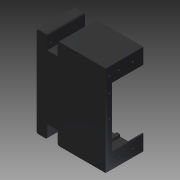
# Autodesk Inventor part: Part1
Saved by Autodesk Inventor 2016 (Build 200138000, 138)
## iProperties
Created: 2015-06-07
Part Number: Part1
Material: ABS Plastic
Document SubType Name: Modeling
Designer: Jufo
Density: 1 g/cm^3
Appearance: Smooth - White
Author: Jufo
Autodesk Inventor part; units mm, degrees
ref_plane "YZ Plane" through (0, 0, 0) normal (1, 0, 0) x (0, 1, 0)
ref_plane "XZ Plane" through (0, 0, 0) normal (0, 1, 0) x (-1, 0, 0)
ref_plane "XY Plane" through (0, 0, 0) normal (0, 0, 1) x (1, 0, 0)
sketch "Sketch1" plane through (0, 0, 0) normal (0, 1, 0) x (-1, 0, 0)
  line L0 (-6.278, 25.2242) -> (-6.278, -144.7758)
  line L1 (-6.278, -144.7758) -> (-26.278, -144.7758)
  line L2 (-26.278, -144.7758) -> (-26.278, -119.7758)
  line L3 (-26.278, -119.7758) -> (-46.278, -119.7758)
  line L4 (-46.278, -119.7758) -> (-46.278, -144.7758)
  line L5 (-46.278, -144.7758) -> (-136.278, -144.7758)
  line L6 (-136.278, -144.7758) -> (-136.278, -134.7758)
  line L7 (-6.278, 25.2242) -> (-26.278, 25.2242)
  line L8 (-26.278, 25.2242) -> (-26.278, 0.2242)
  line L9 (-26.278, 0.2242) -> (-46.278, 0.2242)
  line L10 (-46.278, 0.2242) -> (-46.278, 25.2242)
  line L11 (-46.278, 25.2242) -> (-136.278, 25.2242)
  line L12 (-136.278, 25.2242) -> (-136.278, 15.2242)
  line L13 (-136.278, 15.2242) -> (-136.278, -134.7758)
  point P0 (0, 0)
  dimension "d0" = 170
  dimension "d1" = 20
  dimension "d3" = 20
  dimension "d4" = 90
  dimension "d80" = 20
  dimension "d81" = 150
  dimension "d82" = 10
  dimension "d83" = 10
  dimension "d84" = 90
  dimension "d226" = 25
  dimension "d227" = 25
  dimension "d228" = 25
  constraints: 28 end point, 10 perpendicular, 3 parallel, 1 vertical
  measures "d0" distance of L0.start L0.end
  measures "d1" distance of L0.end L1.end
  measures "d3" distance of L2.end L3.end
  measures "d4" distance of L4.end L5.end
  measures "d80" distance of L0.start L8.start
  measures "d81" distance of L12.end L6.end
  measures "d82" distance of L12.start L12.end
  measures "d83" distance of L5.end L6.end
  measures "d84" distance of L11.start L12.start
  measures "d226" distance of L10.start L11.start
  measures "d227" distance of L3.end L4.end
  measures "d228" distance of L1.end L2.end
extrude "Extrusion1" add sketch "Sketch1" along normal blind 2
sketch "Sketch2" plane through (0, 2, 0) normal (0, 1, 0) x (1, 0, 0)
  line L0 (6.278, 144.7758) -> (6.278, -25.2242) projected
  line L1 (6.278, -25.2242) -> (26.278, -25.2242) projected
  line L2 (26.278, -25.2242) -> (26.278, -0.2242) projected
  line L3 (26.278, -0.2242) -> (46.278, -0.2242) projected
  line L4 (46.278, -0.2242) -> (46.278, -25.2242) projected
  line L5 (46.278, -25.2242) -> (136.278, -25.2242) projected
  line L6 (136.278, -25.2242) -> (136.278, 144.7758) projected
  line L7 (136.278, 144.7758) -> (46.278, 144.7758) projected
  line L8 (46.278, 144.7758) -> (46.278, 119.7758) projected
  line L9 (46.278, 119.7758) -> (26.278, 119.7758) projected
  line L10 (26.278, 119.7758) -> (26.278, 144.7758) projected
  line L11 (26.278, 144.7758) -> (6.278, 144.7758) projected
  line L12 (8.278, 142.7758) -> (24.278, 142.7758)
  line L13 (24.278, 142.7758) -> (24.278, 115.7758)
  line L14 (24.278, 115.7758) -> (48.278, 115.7758)
  line L15 (48.278, 115.7758) -> (48.278, 142.7758)
  line L16 (48.278, 142.7758) -> (134.278, 142.7758)
  line L17 (134.278, 142.7758) -> (134.278, 115.7758)
  line L18 (8.278, 142.7758) -> (8.278, -23.2242)
  line L19 (8.278, -23.2242) -> (24.278, -23.2242)
  line L20 (24.278, -23.2242) -> (24.278, 3.7758)
  line L21 (24.278, 3.7758) -> (48.278, 3.7758)
  line L22 (48.278, 3.7758) -> (48.278, -23.2242)
  line L23 (48.278, -23.2242) -> (134.278, -23.2242)
  line L24 (134.278, -23.2242) -> (134.278, 3.7758)
  line L25 (134.278, 3.7758) -> (136.278, 3.7758)
  line L26 (134.278, 115.7758) -> (136.278, 115.7758)
  point P0 (0, 0)
  dimension "d7" = 2
  dimension "d8" = 2
  dimension "d9" = 2
  dimension "d10" = 4
  dimension "d11" = 2
  dimension "d13" = 2
  dimension "d14" = 2
  dimension "d15" = 4
  dimension "d16" = 2
  dimension "d17" = 2
  dimension "d18" = 2
  dimension "d19" = 2
  dimension "d20" = 2
  dimension "d21" = 27
  dimension "d22" = 27
  constraints: 30 end point, 9 parallel, 6 perpendicular, 2 point on line
  measures "d7" distance between parallel lines of L6 L24
  measures "d8" distance between parallel lines of L5 L23
  measures "d9" distance between parallel lines of L4 L22
  measures "d10" distance between parallel lines of L21 L3
  measures "d11" distance between parallel lines of L0 L18
  measures "d13" distance between parallel lines of L11 L12
  measures "d14" distance between parallel lines of L10 L13
  measures "d15" distance between parallel lines of L9 L14
  measures "d16" distance between parallel lines of L8 L15
  measures "d17" distance between parallel lines of L7 L16
  measures "d18" distance between parallel lines of L6 L17
  measures "d19" distance between parallel lines of L2 L20
  measures "d20" distance between parallel lines of L1 L19
  measures "d21" distance of L16.end L17.end
  measures "d22" distance of L23.end L24.end
extrude "Extrusion2" add sketch "Sketch2" along normal blind 69 contours L11 L10 L9 L8 L7 L6 L26 L17 L16 L15 L14 L13 L12 L18 L19 L20 L21 L22 L23 L24 L25 L5 L4 L3 L2 L1 L0
sketch "Sketch3" plane through (0, 2, 0) normal (0, 1, 0) x (1, 0, 0)
  line L0 (134.278, 3.7758) -> (136.278, 3.7758) projected
  line L1 (136.278, 3.7758) -> (136.278, 115.7758) projected
  line L2 (136.278, 115.7758) -> (134.278, 115.7758) projected
  line L3 (134.278, -23.2242) -> (134.278, 3.7758) projected
  line L4 (134.278, 115.7758) -> (134.278, 3.7758)
  point P0 (0, 0)
  constraints: 2 end point, 1 collinear
extrude "Extrusion3" add sketch "Sketch3" along normal blind 10
sketch "Sketch4" plane through (136.278, 0, 25.2242) normal (1, 0, 0) x (0, 0, -1)
  line L0 (170, 0) -> (0, 0) projected
  line L1 (141, 71) -> (170, 71) projected
  line L2 (29, 12) -> (141, 12) projected
  line L3 (0, 0) -> (0, 71) projected
  line L4 (85, 12) -> (85, 7)
  circle A0 centre (85, 7) radius 1.5
  line L5 (29, 12) -> (44, 12)
  circle A1 centre (44, 7) radius 1.5
  line L6 (141, 12) -> (126, 12)
  circle A2 centre (126, 7) radius 1.5
  line L7 (155.5, 71) -> (155.5, 51)
  line L8 (155.5, 0) -> (155.5, 25)
  circle A3 centre (155.5, 25) radius 1.5
  circle A4 centre (155.5, 51) radius 1.5
  circle A5 centre (14.5, 25) radius 1.5
  circle A6 centre (14.5, 51) radius 1.5
  line L9 (141, 12) -> (141, 71) projected
  line L10 (29, 12) -> (29, 71) projected
  line L11 (170, 0) -> (170, 71) projected
  point P0 (25.2242, 0)
  dimension "d27" = 5
  dimension "d28" = 3
  dimension "d30" = 15
  dimension "d31" = 3
  dimension "d32" = 15
  dimension "d33" = 3
  dimension "d34" = 20
  dimension "d35" = 25
  dimension "d36" = 3
  dimension "d37" = 3
  dimension "d85" = 15
  dimension "d86" = 15
  dimension "d87" = 14.5
  constraints: 10 end point, 7 centre point, 3 coincident, 3 point on line, 2 midpoint, 2 symmetric about line, 1 collinear, 1 parallel, 1 perpendicular, 2 other
  measures "d27" distance of L4.start L4.end
  measures "d28" diameter of A0
  measures "d30" distance of L2.start L5.end
  measures "d31" diameter of A1
  measures "d32" distance of L2.end L6.end
  measures "d33" diameter of A2
  measures "d34" distance of L7.start L7.end
  measures "d35" distance of L8.start L8.end
  measures "d36" diameter of A3
  measures "d37" diameter of A4
  measures "d85" distance from line of L10 A1.centre
  measures "d86" distance from line of L9 A2.centre
  measures "d87" distance from line of L11 A3.centre
extrude "Extrusion4" cut sketch "Sketch4" against normal blind 2
sketch "Sketch5" plane through (46.278, 0, 0.2242) normal (-1, 0, 0) x (0, 0, 1)
  line L0 (0, 0) -> (0, 71) projected
  line L1 (0, 0) -> (0, 7)
  line L2 (0, 7) -> (10, 7)
  circle A0 centre (10, 7) radius 1.6
  point P0 (-0.2242, 0)
  dimension "d40" = 7
  dimension "d41" = 10
  dimension "d42" = 3.2
  constraints: 4 end point, 1 centre point, 1 coincident, 1 perpendicular, 1 point on line
  measures "d40" distance of L0.start L1.end
  measures "d41" distance of L1.end L2.end
  measures "d42" diameter of A0
extrude "Extrusion5" cut sketch "Sketch5" against normal blind 4
sketch "Sketch6" plane through (26.278, 0, 25.2242) normal (1, 0, 0) x (0, 0, -1)
  line L0 (25, 0) -> (25, 71) projected
  line L1 (25, 0) -> (25, 7)
  line L2 (25, 7) -> (15, 7)
  circle A0 centre (15, 7) radius 1.6
  point P0 (25.2242, 0)
  dimension "d45" = 7
  dimension "d46" = 10
  dimension "d47" = 3.2
  constraints: 4 end point, 1 centre point, 1 coincident, 1 perpendicular, 1 point on line
  measures "d45" distance of L0.start L1.end
  measures "d46" distance of L1.end L2.end
  measures "d47" diameter of A0
extrude "Extrusion6" cut sketch "Sketch6" against normal blind 4
sketch "Sketch7" plane through (26.278, 0, -119.7758) normal (1, 0, 0) x (0, 0, -1)
  line L0 (0, 0) -> (0, 71) projected
  line L1 (0, 0) -> (0, 7)
  line L2 (0, 7) -> (10, 7)
  circle A0 centre (10, 7) radius 1.6
  point P0 (-119.7758, 0)
  dimension "d50" = 7
  dimension "d51" = 10
  dimension "d52" = 3.2
  constraints: 4 end point, 1 centre point, 1 coincident, 1 perpendicular, 1 point on line
  measures "d50" distance of L0.start L1.end
  measures "d51" distance of L1.end L2.end
  measures "d52" diameter of A0
extrude "Extrusion7" cut sketch "Sketch7" against normal blind 4
sketch "Sketch8" plane through (46.278, 0, -144.7758) normal (-1, 0, 0) x (0, 0, 1)
  line L0 (25, 0) -> (25, 71) projected
  line L1 (25, 0) -> (25, 7)
  line L2 (25, 7) -> (15, 7)
  circle A0 centre (15, 7) radius 1.6
  point P0 (144.7758, 0)
  dimension "d55" = 7
  dimension "d56" = 10
  dimension "d57" = 3.2
  constraints: 4 end point, 1 centre point, 1 coincident, 1 perpendicular, 1 point on line
  measures "d55" distance of L0.start L1.end
  measures "d56" distance of L1.end L2.end
  measures "d57" diameter of A0
extrude "Extrusion8" cut sketch "Sketch8" against normal blind 4
sketch "Sketch9" plane through (136.278, 0, 25.2242) normal (1, 0, 0) x (0, 0, -1)
  line L0 (170, 0) -> (0, 0) projected
  line L1 (0, 0) -> (0, 71) projected
  line L2 (32, 0) -> (32, 7)
  line L3 (32, 7) -> (15, 7)
  line L4 (148, 0) -> (148, 7)
  line L5 (148, 7) -> (155, 7)
  circle A0 centre (15, 7) radius 1.6
  circle A1 centre (155, 7) radius 1.6
  line L6 (145, 0) -> (145, 71) projected
  line L7 (25, 0) -> (25, 71) projected
  point P0 (25.2242, 0)
  dimension "d60" = 7
  dimension "d63" = 3.2
  dimension "d64" = 3.2
  dimension "d292" = 10
  dimension "d293" = 10
  constraints: 8 end point, 3 perpendicular, 2 centre point, 2 coincident, 2 point on line, 1 parallel
  measures "d60" distance of L2.start L2.end
  measures "d63" diameter of A0
  measures "d64" diameter of A1
  measures "d292" distance from line of L6 A1.centre
  measures "d293" distance from line of A0.centre L7
extrude "Extrusion9" cut sketch "Sketch9" against normal blind 2 contours A0 | A1
sketch "Sketch10" plane through (46.278, 0, -119.7758) normal (0, 0, -1) x (-1, 0, 0)
  line L0 (0, 71) -> (20, 71) projected
  line L1 (0, 0) -> (0, 71) projected
  line L2 (0, 71) -> (0, 64)
  line L3 (0, 64) -> (2.625, 64)
  circle A0 centre (2.625, 64) radius 1.5
  line L4 (10, 71) -> (10, 65.5)
  circle A1 centre (17.375, 64) radius 1.5
  point P0 (46.278, 0)
  dimension "d67" = 7
  dimension "d68" = 2.625
  dimension "d69" = 3
  constraints: 6 end point, 2 centre point, 2 perpendicular, 1 coincident, 1 midpoint, 1 point on line, 1 symmetric about line, 1 other
  measures "d67" distance of L0.start L2.end
  measures "d68" distance of L2.end L3.end
  measures "d69" diameter of A0
extrude "Extrusion10" cut sketch "Sketch10" against normal blind 4
sketch "Sketch11" plane through (26.278, 0, 0.2242) normal (0, 0, 1) x (1, 0, 0)
  line L0 (0, 71) -> (20, 71) projected
  line L1 (0, 0) -> (0, 71) projected
  line L2 (0, 71) -> (0, 64)
  line L3 (0, 64) -> (2.625, 64)
  circle A0 centre (2.625, 64) radius 1.5
  line L4 (10, 71) -> (10, 51.1335)
  circle A1 centre (17.375, 64) radius 1.5
  point P0 (-26.278, 0)
  dimension "d72" = 7
  dimension "d73" = 2.625
  dimension "d74" = 3
  constraints: 6 end point, 2 centre point, 2 perpendicular, 1 coincident, 1 midpoint, 1 point on line, 1 symmetric about line, 1 other
  measures "d72" distance of L0.start L2.end
  measures "d73" distance of L2.end L3.end
  measures "d74" diameter of A0
extrude "Extrusion11" cut sketch "Sketch11" against normal blind 4
sketch "Sketch12" plane through (0, 2, 0) normal (0, 1, 0) x (1, 0, 0)
  line L0 (48.278, -23.2242) -> (134.278, -23.2242) projected
  line L1 (91.278, -23.2242) -> (88.278, -23.2242)
  line L2 (91.278, -23.2242) -> (94.278, -23.2242)
  line L3 (88.278, -23.2242) -> (88.278, -17.2242)
  line L4 (88.278, -17.2242) -> (94.278, -17.2242)
  line L5 (94.278, -17.2242) -> (94.278, -23.2242)
  line L6 (134.278, -23.2242) -> (134.278, 142.7758) projected
  line L7 (48.278, 3.7758) -> (48.278, -23.2242) projected
  line L8 (134.278, 59.7758) -> (89.3363, 59.7758)
  line L9 (88.278, 142.7758) -> (88.278, 136.7758)
  line L10 (88.278, 136.7758) -> (94.278, 136.7758)
  line L11 (94.278, 136.7758) -> (94.278, 142.7758)
  line L12 (134.278, 142.7758) -> (48.278, 142.7758) projected
  line L13 (88.278, 142.7758) -> (94.278, 142.7758)
  line L14 (136.278, -25.2242) -> (136.278, 3.7758) projected
  point P0 (0, 0)
  dimension "d88" = 3
  dimension "d89" = 3
  dimension "d103" = 6
  dimension "d167" = 40
  dimension "d168" = 40
  constraints: 20 end point, 4 symmetric about line, 3 perpendicular, 2 midpoint, 2 point on line, 1 collinear, 1 parallel
  measures "d88" distance of L1.start L1.end
  measures "d89" distance of L1.start L2.end
  measures "d103" distance of L4.end L2.end
  measures "d167" distance between parallel lines of L7 L3
  measures "d168" distance between parallel lines of L6 L5
sketch "Sketch13" plane through (0, 2, 0) normal (0, 1, 0) x (1, 0, 0)
  line L0 (24.278, 142.7758) -> (8.278, 142.7758) projected
  line L1 (8.278, 142.7758) -> (8.278, -23.2242) projected
  line L2 (8.278, -23.2242) -> (24.278, -23.2242) projected
  line L3 (8.278, -23.2242) -> (8.278, -17.2242)
  line L4 (8.278, -17.2242) -> (14.278, -17.2242)
  line L5 (14.278, -17.2242) -> (14.278, -23.2242)
  line L6 (8.278, 142.7758) -> (8.278, 136.7758)
  line L7 (8.278, 136.7758) -> (14.278, 136.7758)
  line L8 (14.278, 136.7758) -> (14.278, 142.7758)
  point P0 (0, 0)
  dimension "d95" = 6
  dimension "d96" = 6
  dimension "d97" = 6
  dimension "d98" = 6
  constraints: 12 end point, 4 perpendicular, 4 point on line
  measures "d95" distance of L1.end L3.end
  measures "d96" distance of L3.end L4.end
  measures "d97" distance of L0.end L6.end
  measures "d98" distance of L6.end L7.end
extrude "Extrusion13" add sketch "Sketch13" along normal blind 67
extrude "Extrusion14" add sketch "Sketch12" along normal blind 67
sketch "Sketch14" plane through (0, 71, 0) normal (0, 1, 0) x (1, 0, 0)
  circle A0 centre (11.278, -20.2242) radius 1.5
  circle A1 centre (11.278, 139.7758) radius 1.5
  circle A2 centre (91.278, 139.7758) radius 1.5
  circle A3 centre (91.278, -20.2242) radius 1.5
  line L0 (48.278, 142.7758) -> (134.278, 142.7758) projected
  line L1 (88.278, 136.7758) -> (94.278, 136.7758) projected
  line L2 (134.278, -23.2242) -> (48.278, -23.2242) projected
  line L3 (24.278, -23.2242) -> (8.278, -23.2242) projected
  line L4 (8.278, -23.2242) -> (8.278, 142.7758) projected
  line L5 (8.278, 136.7758) -> (14.278, 136.7758) projected
  line L6 (88.278, 136.7758) -> (88.278, 142.7758) projected
  line L7 (88.278, -17.2242) -> (88.278, -23.2242) projected
  point P0 (0, 0)
  dimension "d104" = 3
  dimension "d105" = 3
  dimension "d221" = 3
  dimension "d222" = 6
  dimension "d229" = 3
  dimension "d230" = 3
  dimension "d231" = 3
  dimension "d232" = 3
  dimension "d233" = 3
  dimension "d308" = 3
  dimension "d309" = 3
  constraints: 4 centre point
  measures "d104" diameter of A0
  measures "d105" diameter of A2
  measures "d221" distance from line of L1 A2.centre
  measures "d222" distance between parallel lines of L1 L0
  measures "d229" distance from line of L5 A1.centre
  measures "d230" distance from line of L4 A1.centre
  measures "d231" distance from line of L4 A0.centre
  measures "d232" distance from line of L3 A0.centre
  measures "d233" distance from line of L2 A3.centre
  measures "d308" distance from line of L6 A2.centre
  measures "d309" distance from line of L7 A3.centre
extrude "Extrusion15" cut sketch "Sketch14" against normal blind 25
sketch "Sketch22" plane through (24.278, 2, -115.7758) normal (0, 0, 1) x (1, 0, 0)
  line L0 (28, 0) -> (0, 0)
  line L1 (0, 0) -> (0, 69)
  line L2 (14, 0) -> (14, 11)
  line L3 (14, 11) -> (11.5, 11)
  line L4 (11.5, 11) -> (11.5, 16)
  line L5 (11.5, 16) -> (16.5, 16)
  line L6 (16.5, 16) -> (16.5, 11)
  line L7 (16.5, 11) -> (14, 11)
  point P0 (-24.278, -2)
  point P1 (-40.2395, -2)
  dimension "d209" = 11
  dimension "d210" = 2.5
  dimension "d211" = 5
  dimension "d212" = 5
  constraints: 16 end point, 3 parallel, 3 perpendicular, 1 midpoint
  measures "d209" distance of L2.start L2.end
  measures "d210" distance of L2.end L3.end
  measures "d211" distance of L3.end L4.end
  measures "d212" distance of L4.end L5.end
extrude "Extrusion22" cut sketch "Sketch22" against normal blind 4
sketch "Sketch23" plane through (48.278, 2, -3.7758) normal (0, 0, -1) x (-1, 0, 0)
  line L0 (28, 0) -> (0, 0)
  line L1 (0, 0) -> (0, 69)
  line L2 (14, 0) -> (14, 11)
  line L3 (14, 11) -> (11.5, 11)
  line L4 (11.5, 11) -> (11.5, 16)
  line L5 (11.5, 16) -> (16.5, 16)
  line L6 (16.5, 16) -> (16.5, 11)
  line L7 (16.5, 11) -> (14, 11)
  point P0 (48.278, -2)
  point P1 (-40.2395, -2)
  dimension "d215" = 11
  dimension "d216" = 2.5
  dimension "d217" = 5
  dimension "d218" = 5
  constraints: 16 end point, 3 parallel, 3 perpendicular, 1 midpoint
  measures "d215" distance of L2.start L2.end
  measures "d216" distance of L2.end L3.end
  measures "d217" distance of L3.end L4.end
  measures "d218" distance of L4.end L5.end
extrude "Extrusion23" cut sketch "Sketch23" against normal blind 4
sketch "Sketch33" plane through (0, 2, 0) normal (0, 1, 0) x (1, 0, 0)
  circle A0 centre (130.278, 138.7758) radius 1.5
  circle A1 centre (52.278, 138.7758) radius 1.5
  circle A2 centre (130.278, -19.2242) radius 1.5
  circle A3 centre (52.278, -19.2242) radius 1.5
  line L0 (48.278, 142.7758) -> (134.278, 142.7758) projected
  line L1 (134.278, 142.7758) -> (134.278, 115.7758) projected
  line L2 (134.278, -23.2242) -> (126.278, -23.2242)
  line L3 (126.278, -23.2242) -> (126.278, -15.2242)
  line L4 (126.278, -15.2242) -> (134.278, -15.2242)
  line L5 (134.278, -15.2242) -> (134.278, -23.2242)
  line L6 (134.278, 142.7758) -> (126.278, 142.7758)
  line L7 (126.278, 142.7758) -> (126.278, 134.7758)
  line L8 (126.278, 134.7758) -> (134.278, 134.7758)
  line L9 (134.278, 134.7758) -> (134.278, 142.7758)
  line L10 (48.278, 142.7758) -> (56.278, 142.7758)
  line L11 (56.278, 142.7758) -> (56.278, 134.7758)
  line L12 (56.278, 134.7758) -> (48.278, 134.7758)
  line L13 (48.278, 134.7758) -> (48.278, 142.7758)
  line L14 (48.278, -23.2242) -> (56.278, -23.2242)
  line L15 (56.278, -23.2242) -> (56.278, -15.2242)
  line L16 (56.278, -15.2242) -> (48.278, -15.2242)
  line L17 (48.278, -15.2242) -> (48.278, -23.2242)
  point P0 (0, 0)
  point P1 (0, 0)
  dimension "d329" = 78
  dimension "d331" = 4
  dimension "d332" = 158
  dimension "d333" = 158
  dimension "d334" = 78
  dimension "d335" = 4
  dimension "d336" = 8
  dimension "d337" = 8
  dimension "d338" = 8
  dimension "d339" = 8
  dimension "d340" = 8
  dimension "d341" = 8
  dimension "d342" = 8
  dimension "d343" = 8
  constraints: 32 end point, 8 parallel, 4 centre point, 4 horizontal, 4 perpendicular
  measures "d329" distance of A2.centre A3.centre
  measures "d331" distance from line of L0 A0.centre
  measures "d332" distance of A0.centre A2.centre
  measures "d333" distance of A3.centre A1.centre
  measures "d334" distance of A0.centre A1.centre
  measures "d335" distance from line of L1 A0.centre
  measures "d336" distance of L3.end L4.end
  measures "d337" distance of L2.end L3.end
  measures "d338" distance of L8.end L7.end
  measures "d339" distance of L7.end L6.end
  measures "d340" distance of L11.end L12.end
  measures "d341" distance of L10.end L11.end
  measures "d342" distance of L16.end L15.end
  measures "d343" distance of L15.end L14.end
extrude "Extrusion28" add sketch "Sketch33" along normal blind 24
sketch "Sketch34" plane through (0, 2, 0) normal (0, 1, 0) x (1, 0, 0)
  line L0 (134.278, 13.7758) -> (119.278, 13.7758)
  line L1 (134.278, 115.7758) -> (134.278, 3.7758) projected
  line L2 (119.278, 13.7758) -> (119.278, 112.7758)
  line L3 (119.278, 112.7758) -> (88.878, 112.7758)
  line L4 (88.878, 112.7758) -> (88.878, 13.7758)
  line L5 (88.878, 13.7758) -> (119.278, 13.7758)
  line L6 (88.878, 13.7758) -> (88.878, 11.7758)
  line L7 (88.878, 11.7758) -> (121.278, 11.7758)
  line L8 (121.278, 11.7758) -> (121.278, 114.7758)
  line L9 (121.278, 114.7758) -> (86.878, 114.7758)
  line L10 (86.878, 114.7758) -> (86.878, 11.7758)
  line L11 (86.878, 11.7758) -> (88.878, 11.7758)
  line L12 (104.078, 11.7758) -> (104.078, 13.7758)
  line L13 (86.878, 114.7758) -> (54.478, 114.7758)
  line L14 (54.478, 114.7758) -> (54.478, 11.7758)
  line L15 (54.478, 11.7758) -> (86.878, 11.7758)
  line L16 (88.878, 13.7758) -> (86.878, 13.7758)
  line L17 (86.878, 13.7758) -> (56.478, 13.7758)
  line L18 (56.478, 13.7758) -> (56.478, 112.7758)
  line L19 (56.478, 112.7758) -> (86.878, 112.7758)
  line L20 (70.678, 11.7758) -> (70.678, 13.7758)
  line L21 (48.278, 142.7758) -> (134.278, 142.7758) projected
  line L22 (56.478, 13.7758) -> (54.478, 13.7758)
  point P0 (0, 0)
  dimension "d346" = 15
  dimension "d347" = 0
  dimension "d348" = 30.4
  dimension "d349" = 2
  dimension "d350" = 2
  dimension "d352" = 2
  dimension "d353" = 2
  dimension "d354" = 99
  dimension "d355" = 2
  dimension "d356" = 34.4
  dimension "d357" = 32.4
  dimension "d358" = 30.4
  dimension "d359" = 28
  dimension "d360" = 2
  constraints: 42 end point, 8 point on line, 7 perpendicular, 5 parallel, 3 horizontal, 2 midpoint, 2 vertical, 1 collinear
  measures "d346" distance of L0.start L0.end
  measures "d347" distance from line of L1 L0.start
  measures "d348" distance of L2.end L3.end
  measures "d349" distance of L4.end L6.end
  measures "d350" distance between parallel lines of L2 L8
  measures "d352" distance between parallel lines of L3 L9
  measures "d353" distance between parallel lines of L4 L10
  measures "d354" distance of L0.end L2.end
  measures "d355" distance between parallel lines of L7 L5
  measures "d356" distance of L8.end L9.end
  measures "d357" distance of L9.end L13.end
  measures "d358" distance of L16.end L17.end
  measures "d359" distance between parallel lines of L21 L13
  measures "d360" distance between parallel lines of L13 L19
extrude "Extrusion29" add sketch "Sketch34" along normal blind 24 contours L8 L7 L12 L5 L0 | L0 L2 L3 L4 L16 L10 L9 L8 | L10 L19 L18 L22 L14 L13 | L6 L11 L10 L16 | L10 L15 L20 L17
fillet "Fillet1" radius 3 6 edges at (46.278, 35.5, 25.2242) (26.278, 35.5, 25.2242) (6.278, 35.5, 25.2242) (6.278, 35.5, -144.7758) (26.278, 35.5, -144.7758) (46.278, 35.5, -144.7758)
equation "\"d80\" = d1"
equation "\"d8\" = d7"
equation "\"d9\" = d16"
equation "\"d11\" = d8"
equation "\"d13\" = d11"
equation "\"d14\" = d16"
equation "\"d17\" = d11"
equation "\"d18\" = d17"
equation "\"d19\" = d14"
equation "\"d20\" = d7"
body "Solid1"
